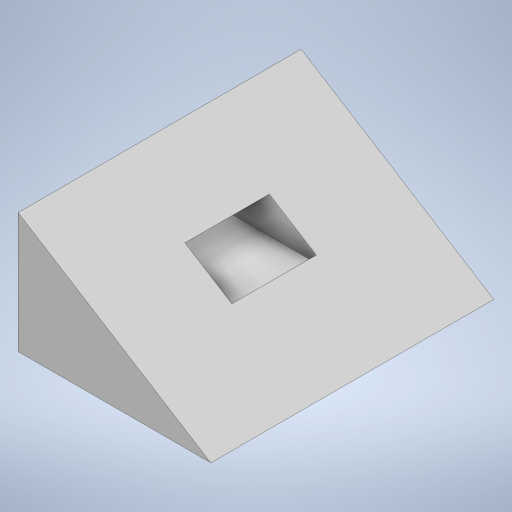
# Autodesk Inventor part: mouseBottom
Saved by Autodesk Inventor 2024.2 (Build 282272000, 272)
## iProperties
Created: 2024-08-04
Part Number: mouseBottom
Material: Generic
Document SubType Name: Modeling
Designer: 875608
Density: 1 g/cm^3
Appearance: Default
Author: 875608
Autodesk Inventor part; units mm, degrees
ref_plane "YZ Plane" through (0, 0, 0) normal (1, 0, 0) x (0, 1, 0)
ref_plane "XZ Plane" through (0, 0, 0) normal (0, 1, 0) x (-1, 0, 0)
ref_plane "XY Plane" through (0, 0, 0) normal (0, 0, 1) x (1, 0, 0)
sketch "Sketch1" plane through (0, 0, 0) normal (0, 0, 1) x (1, 0, 0)
  line L0 (0, 0) -> (0, 20)
  line L1 (0, 0) -> (32, 0)
  line L2 (32, 0) -> (0, 20)
  dimension "d0" = 20
  dimension "d1" = 32
  constraints: 6 end point, 1 horizontal, 1 vertical
  measures "d0" distance of L0.start L0.end
  measures "d1" distance of L0.start L1.end
extrude "Extrusion1" add sketch "Sketch1" along normal blind 47
sketch "Sketch2" plane through (0, 0, 0) normal (-1, 0, 0) x (0, 0, 1)
  line L0 (0, 0) -> (47, 0) projected
  line L1 (0, 20) -> (0, 0) projected
  line L2 (0, 0) -> (0, 20)
  line L3 (0, 20) -> (47, 20) projected
  line L4 (0, 20) -> (47, 20)
  line L5 (23.5, 13) -> (16.5, 13)
  line L6 (16.5, 13) -> (30.5078, 13)
  line L7 (30.5078, 13) -> (30.5078, 6.9967)
  line L8 (30.5078, 6.9967) -> (16.5, 6.9967)
  line L9 (16.5, 6.9967) -> (16.5, 13)
  dimension "d5" = 7
  dimension "d6" = 15.24
  constraints: 14 end point, 2 parallel, 2 perpendicular, 1 horizontal, 1 vertical
  measures "d5" distance of L5.start L5.end
  measures "d6" distance of L5.end L7.end
extrude "Extrusion2" cut sketch "Sketch2" against normal blind 19
body "Solid1"
